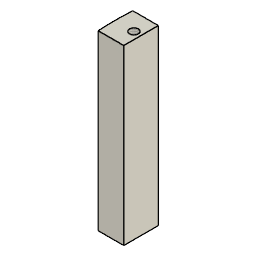
pillars (Autodesk Fusion 360 design; units mm, degrees)
Autodesk Fusion 360 part; units mm, degrees
sketch "Sketch1" plane through (0, 0, 0) normal (0, 0, 1) x (1, 0, 0)
  line L0 (-84.05, 0) -> (-80.45, 0) construction
  line L1 (-84.05, 0) -> (-82, 0) construction
  line L2 (-84.05, 0) -> (-82.5, 0) construction
  circle A0 centre (-82.5, 0) radius 1.55
  line L3 (-80.95, 0) -> (-80.45, 0)
  line L4 (-80.45, 0) -> (-80.45, 2)
  line L5 (-80.45, 2) -> (-84.9765, 2)
  line L6 (-80.45, -2) -> (-84.9765, -2)
  line L7 (-80.45, 0) -> (-80.45, -2)
  arc A1 (-84.9765, 2) -> (-84.9765, -2) centre (0, 0) ccw
  dimension "d6" = 3.1
  dimension "d7" = 0.5
  dimension "d8" = 2
  constraint parallel L1 L2
  constraint coincident L2.end A0.centre
  constraint coincident L0 L3.start
  constraint coincident A0 L3.start
  constraint parallel L0 L3
  constraint perpendicular L0 L4
  constraint perpendicular L4 L5
  constraint symmetric L0 L4.end L6.start
  constraint symmetric L0 L5.end L6.end
  constraint coincident A0 L0.start
  measures "d6" diameter of A0
  measures "d7" distance of L3.start L0.end
  measures "d8" distance of L0.end L4.end
extrude "Extrude1" add sketch "Sketch1" along normal blind 50
thread "Thread1" "ISO Metric profile 3.0 M3x0.5 M3x0.5 6H" major diameter 3.086 minor diameter 2.529 pitch 0.5 angle 60 resizes the face on face at (-83.5823, 1.1096, 33.3333)
move_face "OffsetFaces1" offset 3 3 faces at (-81.9588, 2, 33.3333) (-84.9858, 1.5556, 16.6667) (-81.9588, -2, 33.3333)
